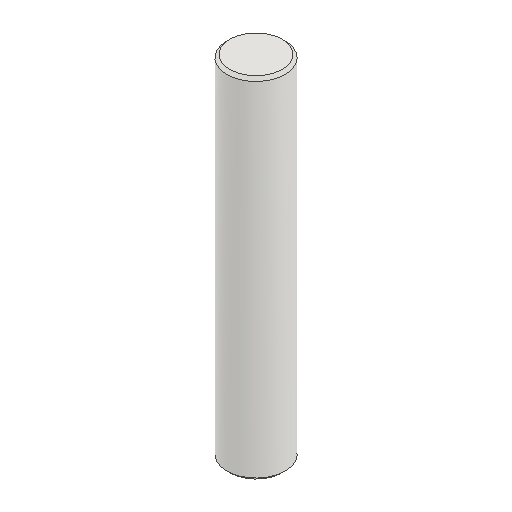
# Autodesk Inventor part: EJE
Saved by Autodesk Inventor 2025 (Build 290162000, 162)
## iProperties
Created: 2026-02-06
Part Number: EJE
Material: Genérico
Document SubType Name: Modeling
Designer: HP
Density: 1 g/cm^3
Appearance: Acero
Author: HP
Autodesk Inventor part; units mm, degrees
ref_plane "YZ Plane" through (0, 0, 0) normal (1, 0, 0) x (0, 1, 0)
ref_plane "XZ Plane" through (0, 0, 0) normal (0, 1, 0) x (-1, 0, 0)
ref_plane "XY Plane" through (0, 0, 0) normal (0, 0, 1) x (1, 0, 0)
sketch "Boceto1" plane through (0, 0, 0) normal (0, 1, 0) x (-1, 0, 0)
  circle A0 centre (0.3797, 0) radius 5
  point P0 (0, 0)
  dimension "d0" = 10
  constraints: 1 centre point
  measures "d0" diameter of A0
extrude "Extrusión1" add sketch "Boceto1" along normal blind 60
chamfer "Chaflán1" distance 0.5 angle 45 1 edges at (4.6203, 60, 0)
chamfer "Chaflán2" distance 0.5 angle 45 1 edges at (4.6203, 0, 0)
